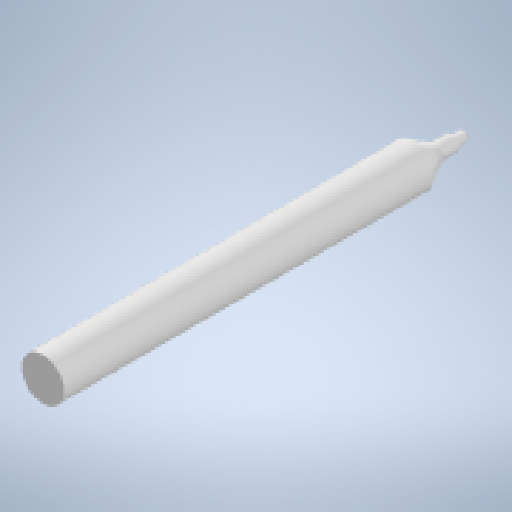
# Autodesk Inventor part: marker
Saved by Autodesk Inventor 2024 (Build 280153000, 153)
## iProperties
Created: 2026-02-15
Part Number: marker
Material: Generic
Document SubType Name: Modeling
Designer: SEMEN
Density: 1 g/cm^3
Appearance: Default
Author: SEMEN
Autodesk Inventor part; units mm, degrees
ref_plane "YZ Plane" through (0, 0, 0) normal (1, 0, 0) x (0, 1, 0)
ref_plane "XZ Plane" through (0, 0, 0) normal (0, 1, 0) x (-1, 0, 0)
ref_plane "XY Plane" through (0, 0, 0) normal (0, 0, 1) x (1, 0, 0)
sketch "Sketch1" plane through (0, 0, 0) normal (1, 0, 0) x (0, 1, 0)
  line L0 (0, 0) -> (0, -131.8102)
  line L1 (0, 0) -> (6.5551, 0)
  line L2 (6.5551, 0) -> (6.5551, -114.3933)
  line L3 (6.5551, -114.3933) -> (5.4607, -114.3933)
  line L4 (5.4607, -114.3933) -> (5.4607, -116.2052)
  line L5 (5.4607, -116.2052) -> (3.8817, -116.2052)
  line L6 (3.8817, -116.2052) -> (3.8817, -118.5274)
  line L7 (3.8817, -118.5274) -> (2.3955, -121.4998)
  line L8 (2.3955, -121.4998) -> (2.3955, -126.4228)
  line L9 (2.3955, -126.4228) -> (1.6524, -126.4228)
  line L10 (1.6524, -126.4228) -> (1.6524, -129.8596)
  line L11 (1.6524, -129.8596) -> (0, -131.8102)
  constraints: 24 end point, 6 perpendicular, 2 horizontal, 1 parallel, 1 vertical
revolve "Revolution1" add sketch "Sketch1" angle 360 about axis through (0, 0, 0) along (0, 0, -1)
body "Solid1"
